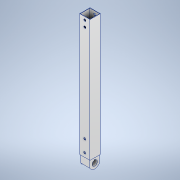
# Autodesk Inventor part: Brazo
Saved by Autodesk Inventor 2022 (Build 260153000, 153)
## iProperties
Created: 2021-10-22
Part Number: Brazo
Material: Aluminum 6061
Document SubType Name: Modeling
Designer: juanp
Density: 2.7 g/cm^3
Appearance: Aluminum - Flat
Author: juanp
Autodesk Inventor part; units mm, degrees
ref_plane "YZ Plane" through (0, 0, 0) normal (1, 0, 0) x (0, 1, 0)
ref_plane "XZ Plane" through (0, 0, 0) normal (0, 1, 0) x (-1, 0, 0)
ref_plane "XY Plane" through (0, 0, 0) normal (0, 0, 1) x (1, 0, 0)
sketch "Sketch1" plane through (0, 0, 0) normal (0, 1, 0) x (-1, 0, 0)
  line L0 (12.7, 12.7) -> (-12.7, 12.7)
  line L1 (-12.7, 12.7) -> (-12.7, -12.7)
  line L2 (-12.7, -12.7) -> (12.7, -12.7)
  line L3 (12.7, -12.7) -> (12.7, 12.7)
  line L4 (12.7, 12.7) -> (-12.7, -12.7) construction
  line L5 (-12.7, 12.7) -> (12.7, -12.7) construction
  line L6 (-11.7, -11.7) -> (11.7, -11.7)
  line L7 (11.7, -11.7) -> (11.7, 11.7)
  line L8 (11.7, 11.7) -> (-11.7, 11.7)
  line L9 (-11.7, 11.7) -> (-11.7, -11.7)
  line L10 (-11.7, -11.7) -> (11.7, 11.7) construction
  line L11 (11.7, -11.7) -> (-11.7, 11.7) construction
  point P0 (0, 0)
  dimension "d0" = 25.4
  dimension "d1" = 1
  constraints: 24 end point, 4 midpoint, 4 parallel, 3 perpendicular, 2 horizontal, 1 point on line
  measures "d0" distance of L2.end L0.start
  measures "d1" distance between parallel lines of L3 L7
extrude "Extrusion1" add sketch "Sketch1" along normal blind 325
ref_plane "Work Plane1" through (-12.7, 325, 12.7) normal (0, 0.7504226, 0.6609583) x (1, 0, 0)
sketch "Sketch4" plane through (0, 0, 0) normal (0, -1, 0) x (1, 0, 0)
  line L0 (11.5, -11.5) -> (-11.5, -11.5)
  line L1 (-11.5, -11.5) -> (-11.5, 11.5)
  line L2 (-11.5, 11.5) -> (11.5, 11.5)
  line L3 (11.5, 11.5) -> (11.5, -11.5)
  line L4 (11.5, -11.5) -> (-11.5, 11.5) construction
  line L5 (-11.5, -11.5) -> (11.5, 11.5) construction
  line L6 (11.7, 11.7) -> (-11.7, 11.7) projected
  point P0 (0, 0)
  dimension "d9" = 0.2
  constraints: 12 end point, 2 midpoint, 2 parallel, 2 perpendicular, 1 horizontal
  measures "d9" distance between parallel lines of L6 L2
extrude "Extrusion3" add sketch "Sketch4" against normal blind 75 separate body
sketch "Sketch6" plane through (0, 0, 0) normal (0, -1, 0) x (1, 0, 0)
  line L0 (12.7, 12.7) -> (12.7, -12.7) projected
  line L1 (-12.7, 12.7) -> (12.7, 12.7) projected
  line L2 (-12.7, -12.7) -> (-12.7, 12.7) projected
  line L3 (12.7, -12.7) -> (-12.7, -12.7) projected
  line L4 (11.7, -11.7) -> (11.7, 11.7) projected
  line L5 (-11.7, -11.7) -> (11.7, -11.7) projected
  line L6 (-11.7, 11.7) -> (-11.7, -11.7) projected
  line L7 (11.7, 11.7) -> (-11.7, 11.7) projected
  point P0 (0, 0)
extrude "Extrusion5" cut sketch "Sketch6" against normal blind 25.4 bodies 1
sketch "Sketch5" plane through (-12.7, 0, -12.7) normal (-1, 0, 0) x (0, 0, 1)
  circle A0 centre (12.7, 12.7) radius 12.7
  line L0 (25.4, 0) -> (25.4, 325) projected
  line L1 (0, 0) -> (25.4, 0) projected
  line L2 (0, 0) -> (0, 325) projected
  circle A1 centre (12.7, 12.7) radius 6.35
  line L3 (14.2, 20.4703) -> (11.2, 20.4703)
  line L4 (11.2, 20.4703) -> (11.2, 17.4703)
  line L5 (11.2, 17.4703) -> (14.2, 17.4703)
  line L6 (14.2, 17.4703) -> (14.2, 20.4703)
  line L7 (12.7, 17.4703) -> (12.7, 19.05) construction
  point P0 (12.7, 0)
  point P1 (17.3368, 8.3615)
  point P2 (0, 12.7)
  point P3 (12.7, 0)
  point P4 (25.4, 12.7)
  point P5 (14.2, 18.8703)
  point P6 (11.2, 18.8703)
  dimension "d32" = 1.4
  dimension "d33" = 3
  dimension "d34" = 12.7
  constraints: 10 end point, 3 point on circle, 3 tangent, 2 centre point, 2 coincident, 2 parallel, 2 perpendicular, 1 horizontal, 1 line through centre, 1 midpoint, 1 point on line, 1 vertical
  measures "d32" distance of L5.end point (14.2, 18.87)
  measures "d33" distance of L4.end L5.end
  measures "d34" diameter of A1
extrude "Extrusion4" cut sketch "Sketch5" against normal through all contours L0 L1 A0 | A0 L1 L2 | A1 L4 L5 L6 | L6 L5 L4 A1 | A1 L4 L3 L6 bodies 1 2
sketch "Sketch7" plane through (-12.7, 325, 12.7) normal (0, 0, 1) x (1, 0, 0)
  line L0 (12.7, -289.6) -> (12.7, -260) construction
  line L1 (12.7, -260) -> (12.7, -250) construction
  line L2 (12.7, -289.6) -> (12.7, -299.6) construction
  circle A0 centre (12.7, -260) radius 2.65
  circle A1 centre (12.7, -289.6) radius 2.65
  line L3 (1.2, -250) -> (24.2, -250) projected
  line L4 (0, -299.6) -> (25.4, -299.6) projected
  dimension "d20" = 5.3
  dimension "d21" = 10
  constraints: 7 end point, 2 centre point, 2 coincident, 2 collinear, 2 midpoint, 1 equal radius, 1 vertical
  measures "d20" diameter of A1
  measures "d21" distance of L1.end L0.end
extrude "Extrusion6" cut sketch "Sketch7" against normal through all bodies 1 2
sketch "Sketch8" plane through (-12.7, 325, 12.7) normal (0, 0, 1) x (1, 0, 0)
  line L0 (25.4, 0) -> (0, 0) projected
  line L1 (25.4, -299.6) -> (25.4, 0) projected
  line L2 (0, -299.6) -> (0, 0) projected
  line L3 (12.7, 0) -> (12.7, -7.5) construction
  line L4 (12.7, -7.5) -> (12.7, -22.5) construction
  circle A0 centre (12.7, -7.5) radius 2.65
  circle A1 centre (12.7, -22.5) radius 2.65
  point P0 (12.7, -325)
  dimension "d26" = 7.5
  dimension "d27" = 15
  dimension "d28" = 5.3
  dimension "d29" = 5.3
  constraints: 4 end point, 2 centre point, 2 coincident, 1 midpoint, 1 point on line, 1 vertical
  measures "d26" distance of L3.start L3.end
  measures "d27" distance of L3.end L4.end
  measures "d28" diameter of A0
  measures "d29" diameter of A1
extrude "Extrusion7" cut sketch "Sketch8" against normal through all bodies 1
body "Solid1"
body "Solid2"
